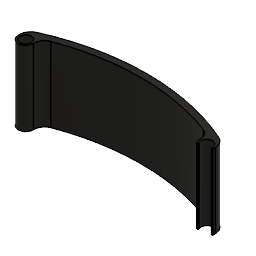
Battery Door v1 (Autodesk Fusion 360 design; units mm, degrees)
part number: 2026-03-17-16-00-33-263
Autodesk Fusion 360 part; units mm, degrees
note: some values were not read from the file. Set by a fixed rule: which sketch regions a step uses.
sketch "Sketch1" plane through (0, 0, 0) normal (0, 1, 0) x (1, 0, 0)
  circle A0 centre (-42.426, 90.51) radius 1.65
  circle A1 centre (-42.426, 90.51) radius 2.65
  circle A2 centre (-42.426, 90.51) radius 3.5
  line L0 (-45.8757, 91.1011) -> (-45.8757, 94.448)
  circle A3 centre (42.426, 90.51) radius 3.5
  circle A4 centre (42.426, 90.51) radius 2.65
  circle A5 centre (42.426, 90.51) radius 1.65
  line L1 (45.8757, 91.1011) -> (45.8757, 94.448)
  arc A6 (45.8757, 94.448) -> (-45.8757, 94.448) centre (0, 0) ccw
  arc A7 (40.6735, 93.5396) -> (-40.6735, 93.5396) centre (0, 0) ccw
  line L2 (42.426, 90.51) -> (45.8757, 91.1011) construction
  line L3 (42.426, 90.51) -> (38.9763, 89.9189) construction
  line L4 (42.426, 90.51) -> (39.559, 88.5025)
  line L5 (42.426, 90.51) -> (45.926, 90.51) construction
  line L6 (42.426, 90.51) -> (41.9784, 93.1219) construction
  line L7 (42.426, 90.51) -> (45.8067, 89.6041)
  line L8 (42.426, 90.51) -> (38.926, 90.51) construction
  dimension "d5" = 3.3
  dimension "d7" = 5.3
  dimension "d8" = 7
  dimension "d18" = 145
  dimension "d19" = 165
  constraint coincident A6.centre A7.centre
  constraint concentric A1 A2
  constraint coincident A2 L0.start
  constraint vertical L0
  constraint coincident A3 A7.start
  constraint coincident A2 A7.end
  constraint coincident A3.centre A4.centre
  constraint coincident A3 L3.end
  constraint parallel L2 L3
  constraint horizontal L5
  constraint coincident A3 L4.end
  constraint coincident A4 L6.end
  constraint perpendicular L2 L6
  constraint horizontal L8
  constraint coincident A3 L7.end
  measures "d5" diameter of A0
  measures "d7" diameter of A1
  measures "d8" diameter of A2
  measures "d18" angle of L4 L5
  measures "d19" angle of L7 L8
extrude "Extrude1" add sketch "Sketch1" along normal blind 35 contours A2 | A2 L0 A3 L1 A6 A7 | A3 A4 L4 L7 picked at (41.0291, 93.4004)
fillet "Fillet1" radius 5.5 1 edges at (-45.8757, 17.5, -94.448)
fillet "Fillet2" radius 5.5 1 edges at (45.8757, 17.5, -94.448)
fillet "Fillet3" radius 5 2 edges at (-40.6735, 17.5, -93.5396) (40.6735, 17.5, -93.5396)
fillet "Fillet4" radius 0.3 4 edges at (40.2552, 17.5, -88.99) (39.559, 17.5, -88.5025) (45.8067, 17.5, -89.6041) (44.9857, 17.5, -89.8241)
sketch "Sketch2" plane through (0, 0, 0) normal (0, 0, 1) x (1, 0, 0)
  line L0 (39.6806, 1.3525) -> (-39.8666, 1.3525) construction
  line L1 (-39.8666, 1.3525) -> (-39.8666, 32.2382) construction
  line L2 (-39.8666, 32.2382) -> (39.6806, 32.2382) construction
  line L3 (39.6806, 32.2382) -> (39.6806, 1.3525) construction
  dimension "d22" = 14
  text T0 "Hyperion" font "Arial" height 14 align centre middle in box 79.5472 x 30.8856 at (39.6806, 1.3525) x (-1, 0) y (0, 1) spacing 1
extrude "Extrude2" cut sketch "Sketch2" along normal blind 1.5 from the near side of the face at (38.1078, 11.6667, -97.8407) text T0
equation "d23 = 'Hyperion'"
